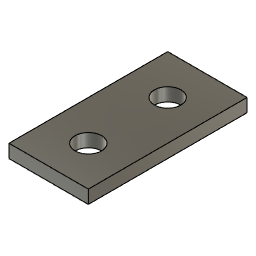
geral (Autodesk Fusion 360 archive; units mm, degrees)
design "Base 1"
Autodesk Fusion 360 part; units mm, degrees
sketch "Esboço3" plane through (0, 0, 0) normal (0, 0, 1) x (1, 0, 0)
box "Primitiva de caixa2" add length 60 width 30 height 5 placed x (0, 1, 0) y (-1, 0, 0) z (0, 0, 1) at (30, 0, 0)
cylinder "Cilindro primitivo2" cut diameter 10 height -35 placed x (1, 0, 0) y (0, 1, 0) z (0, 0, 1) at (15, 15, 5)
cylinder "Cilindro primitivo3" cut diameter 10 height -8 placed x (1, 0, 0) y (0, 1, 0) z (0, 0, 1) at (15, 45, 5)

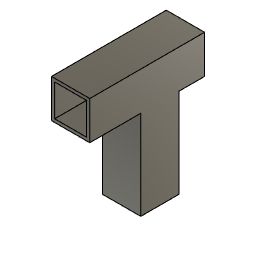
design "suporte motor 90º"
Autodesk Fusion 360 part; units mm, degrees
form "Forma1" [no effect]
box "Primitiva de caixa1" add length 30 width 30 height 70 placed x (0, -1, 0) y (1, 0, 0) z (0, 0, 1) at (-30, 0, 0)
box "Primitiva de caixa2" add length 30 width 30 height -70 placed x (0, 0, 1) y (1, 0, 0) z (0, 1, 0) at (-30, 0, 70)
box "Primitiva de caixa3" add length 30 width 30 height 20 placed x (0, 0, -1) y (-1, 0, 0) z (0, 1, 0) at (0, 0, 100)
shell "Casca1" thickness 5 removed faces 0 bodies 1
box "Primitiva de caixa4" cut length 25 width 25 height -85 placed x (0, 0, 1) y (-1, 0, 0) z (0, -1, 0) at (-2.5, -70, 72.5)
box "Primitiva de caixa5" cut length 10 width 10 height -6 placed x (0, 1, 0) y (1, 0, 0) z (0, 0, -1) at (-20, 5, 70)
cylinder "Cilindro primitivo1" cut diameter 10 height -63 placed x (0, 1, 0) y (1, 0, 0) z (0, 0, -1) at (-15, -15, 0)
